# Autodesk Inventor part: ADUM5000ARWZ
Saved by Autodesk Inventor 2016 (Build 200138000, 138)
## iProperties
Created: 2016-04-08
Part Number: ADUM5000ARWZ
Material: Generic
Document SubType Name: Modeling
Designer: Paschalis
Density: 1 g/cm^3
Appearance: SOIC127P1032X265-16N, ADUM5000ARWZ
Author: Paschalis
Autodesk Inventor part; units mm, degrees
ref_plane "YZ Plane" through (0, 0, 0) normal (1, 0, 0) x (0, 1, 0)
ref_plane "XZ Plane" through (0, 0, 0) normal (0, 1, 0) x (-1, 0, 0)
ref_plane "XY Plane" through (0, 0, 0) normal (0, 0, 1) x (1, 0, 0)
sketch "SOIC127P1032X265-16N, ADUM5000ARWZ_7" plane through (0, 0, 0) normal (0, 0, 1) x (1, 0, 0)
  line L0 (-5.334, 5.2578) -> (5.9944, 5.2578)
  line L1 (5.9944, 5.2578) -> (5.9944, -5.2578)
  line L2 (5.9944, -5.2578) -> (-5.334, -5.2578)
  line L3 (-5.334, -5.2578) -> (-5.334, 5.2578)
  constraints: 8 end point
extrude "Extrusion1" add sketch "SOIC127P1032X265-16N, ADUM5000ARWZ_7" along normal blind 1
body "Solid1"
